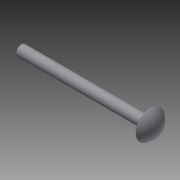
# Autodesk Inventor part: 3in_bolt_for_belt_tightening
Saved by Autodesk Inventor 2015 (Build 190159000, 159)
## iProperties
Created: 2017-03-25
Part Number: 3in_bolt_for_belt_tightening
Material: Generic
Document SubType Name: Modeling
Designer: Guy
Density: 1 g/cm^3
Appearance: Default
Author: Guy
Autodesk Inventor part; units mm, degrees
ref_plane "YZ Plane" through (0, 0, 0) normal (1, 0, 0) x (0, 1, 0)
ref_plane "XZ Plane" through (0, 0, 0) normal (0, 1, 0) x (-1, 0, 0)
ref_plane "XY Plane" through (0, 0, 0) normal (0, 0, 1) x (1, 0, 0)
sketch "Sketch1" plane through (0, 0, 0) normal (0, 0, 1) x (1, 0, 0)
  line L0 (0, 0) -> (0, 3.175)
  line L1 (0, 3.175) -> (76.2, 3.175)
  line L2 (0, 0) -> (81.2, 0)
  line L3 (76.2, 3.175) -> (76.2, 8.5)
  arc A0 (81.2, 0) -> (76.2, 8.5) centre (71.475, 0) ccw
  dimension "d0" = 3.175
  dimension "d1" = 76.2
  dimension "d3" = 5
  dimension "d4" = 8.5
  constraints: 8 end point, 2 point on circle, 2 vertical, 1 centre point, 1 horizontal, 1 perpendicular, 1 point on line
  measures "d0" distance between parallel lines of L2 L1
  measures "d1" distance of L0.end L1.end
  measures "d3" distance from line of L3 L2.end
  measures "d4" distance from line of L2 L3.end
revolve "Revolution1" add sketch "Sketch1" angle 360 about axis through (0, 0, 0) along (1, 0, 0)
body "Solid1"
